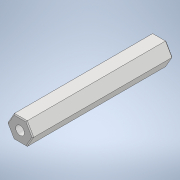
# Autodesk Inventor part: spacers
Saved by Autodesk Inventor 2022 (Build 260153000, 153)
## iProperties
Created: 2021-09-20
Part Number: spacers
Material: Generic
Document SubType Name: Modeling
Designer: TakeHomePC
Density: 1 g/cm^3
Appearance: Default
Author: TakeHomePC
Autodesk Inventor part; units mm, degrees
ref_plane "YZ Plane" through (0, 0, 0) normal (1, 0, 0) x (0, 1, 0)
ref_plane "XZ Plane" through (0, 0, 0) normal (0, 1, 0) x (-1, 0, 0)
ref_plane "XY Plane" through (0, 0, 0) normal (0, 0, 1) x (1, 0, 0)
sketch "Sketch1" plane through (0, 0, 0) normal (0, 0, 1) x (1, 0, 0)
  circle A0 centre (0, 0) radius 2.5
  line L0 (-7.3323, 0) -> (-3.6662, 6.35)
  line L1 (-3.6662, 6.35) -> (3.6662, 6.35)
  line L2 (3.6662, 6.35) -> (7.3323, 0)
  line L3 (7.3323, 0) -> (3.6662, -6.35)
  line L4 (3.6662, -6.35) -> (-3.6662, -6.35)
  line L5 (-3.6662, -6.35) -> (-7.3323, 0)
  dimension "d0" = 5
  dimension "d1" = 12.7
  constraints: 12 end point, 2 coincident, 1 centre point, 13 other
  measures "d0" diameter of A0
  measures "d1" distance between parallel lines of L4 L1
extrude "Extrusion1" add sketch "Sketch1" along normal blind 79.835
chamfer "Chamfer1" distance 0.5 angle 45 12 edges at (0, -6.35, 0) (-5.4993, -3.175, 0) (-5.4993, 3.175, 0) (0, 6.35, 0) (5.4993, 3.175, 0) (5.4993, -3.175, 0) (0, -6.35, 79.835) (5.4993, -3.175, 79.835) (5.4993, 3.175, 79.835) (0, 6.35, 79.835) (-5.4993, 3.175, 79.835) (-5.4993, -3.175, 79.835)
body "Solid1"
